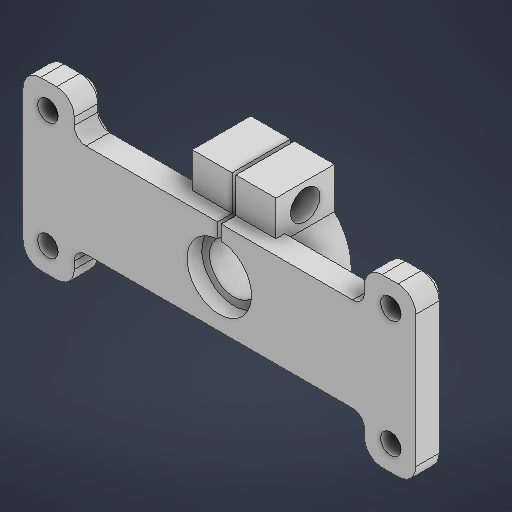
# Autodesk Inventor part: EndEffector_Holder_TEST
Saved by Autodesk Inventor 2025.2 (Build 292293000, 293)
## iProperties
Created: 2025-07-03
Part Number: EndEffector_Holder_TEST
Material: Generic
Document SubType Name: Modeling
Designer: Tiago
Density: 1 g/cm^3
Appearance: Default
Author: Tiago
Autodesk Inventor part; units mm, degrees
note: some values were not read from the file. Chosen so that the rebuilt part matches the saved one: sides of "Extrusion4".
ref_plane "YZ Plane" through (0, 0, 0) normal (1, 0, 0) x (0, 1, 0)
ref_plane "XZ Plane" through (0, 0, 0) normal (0, 1, 0) x (-1, 0, 0)
ref_plane "XY Plane" through (0, 0, 0) normal (0, 0, 1) x (1, 0, 0)
sketch "Sketch1" plane through (0, 0, 0) normal (0, 0, 1) x (1, 0, 0)
  line L0 (33.5, -11.25) -> (33.5, 11.25)
  line L1 (-33.5, 11.25) -> (-33.5, -11.25)
  circle A0 centre (-29.25, 10) radius 1.75
  circle A1 centre (29.25, 10) radius 1.75
  circle A2 centre (-29.25, -10) radius 1.75
  circle A3 centre (29.25, -10) radius 1.75
  circle A4 centre (0, 0) radius 5.5
  arc A5 (-30.5, 14.25) -> (-33.5, 11.25) centre (-30.5, 11.25) ccw
  arc A6 (-33.5, -11.25) -> (-30.5, -14.25) centre (-30.5, -11.25) ccw
  arc A7 (30.5, -14.25) -> (33.5, -11.25) centre (30.5, -11.25) ccw
  arc A8 (33.5, 11.25) -> (30.5, 14.25) centre (30.5, 11.25) ccw
  line L2 (-24.75, 10) -> (-24.75, 11.25)
  line L3 (24.75, 10) -> (24.75, 11.25)
  line L4 (30.5, 14.25) -> (27.75, 14.25)
  line L5 (-27.75, 14.25) -> (-30.5, 14.25)
  line L6 (-30.5, -14.25) -> (-27.75, -14.25)
  line L7 (27.75, -14.25) -> (30.5, -14.25)
  arc A9 (27.75, 14.25) -> (24.75, 11.25) centre (27.75, 11.25) ccw
  arc A10 (24.75, -11.25) -> (27.75, -14.25) centre (27.75, -11.25) ccw
  arc A11 (-27.75, -14.25) -> (-24.75, -11.25) centre (-27.75, -11.25) ccw
  arc A12 (-24.75, 11.25) -> (-27.75, 14.25) centre (-27.75, 11.25) ccw
  circle A13 centre (0, 0) radius 4.2
  line L8 (0, 0) -> (0, 1.4867) construction
  line L9 (-22.75, 8) -> (22.75, 8)
  line L10 (-22.75, -8) -> (22.75, -8)
  arc A14 (22.75, 8) -> (24.75, 10) centre (22.75, 10) ccw
  arc A15 (-24.75, 10) -> (-22.75, 8) centre (-22.75, 10) ccw
  line L11 (-24.75, -11.25) -> (-24.75, -10)
  line L12 (24.75, -11.25) -> (24.75, -10)
  arc A16 (24.75, -10) -> (22.75, -8) centre (22.75, -10) ccw
  arc A17 (-22.75, -8) -> (-24.75, -10) centre (-22.75, -10) ccw
  point P0 (-33.5, 0)
  point P1 (33.5, 0)
  point P2 (-24.75, -8)
  point P3 (24.75, -8)
  dimension "d0" = 58.5
  dimension "d1" = 3.5
  dimension "d2" = 3.5
  dimension "d3" = 20
  dimension "FF" = 3.5
  dimension "d5" = 3.5
  dimension "d7" = 67
  dimension "d8" = 29.25
  dimension "d9" = 10
  dimension "d10" = 11
  dimension "d11" = 3
  dimension "d12" = 4.5
  dimension "d13" = 4.5
  dimension "d14" = 3
  dimension "d15" = 33.5
  dimension "d16" = 28.5
  dimension "d17" = 8.4
  dimension "d27" = 2.5
  dimension "d28" = 8
  dimension "d29" = 2
  dimension "d30" = 2
  constraints: 28 tangent, 26 end point, 24 point on circle, 18 centre point, 9 perpendicular, 8 equal radius, 8 point on line, 5 horizontal alignment, 5 parallel, 2 coincident, 2 horizontal, 2 midpoint, 2 vertical, 2 vertical alignment
  measures "d0" distance of A1.centre A0.centre
  measures "d1" diameter of A1
  measures "d2" diameter of A0
  measures "d3" distance of A0.centre A2.centre
  measures "FF" diameter of A2
  measures "d5" diameter of A3
  measures "d7" distance between parallel lines of L0 L1
  measures "d8" horizontal distance of point (0, 0) A1.centre
  measures "d9" vertical distance of point (0, 0) A1.centre
  measures "d10" diameter of A4
  measures "d11" radius of A5
  measures "d12" distance from line of A2.centre L2
  measures "d13" distance from line of A1.centre L3
  measures "d14" radius of A9
  measures "d15" distance from line of point (0, 0) L0
  measures "d16" distance between parallel lines of L7 L4
  measures "d17" diameter of A13
  measures "d27" distance edge to line of A4 L10
  measures "d28" distance from line of L9 point (0, 0)
  measures "d29" radius of A14
  measures "d30" radius of A16
extrude "Extrusion1" add sketch "Sketch1" along normal blind 5 contours A7 L7 A10 L12 A16 L10 A17 L11 A11 L6 A6 L1 A5 L5 A12 L2 A15 L9 A14 L3 A9 L4 A8 L0
extrude "Extrusion2" add sketch "Sketch1" along normal blind 2.5 contours A4
sketch "Sketch2" plane through (0, 0, 0) normal (0, 0, -1) x (-1, 0, 0)
  circle A0 centre (0, 0) radius 4.2
  circle A1 centre (0, 0) radius 10
  line L0 (0, -10) -> (0, 14) construction
  line L1 (0, 14) -> (0, 9.5) construction
  line L2 (0, 9.5) -> (3.1225, 9.5) construction
  line L3 (3.1225, 7) -> (3.1225, 12)
  line L4 (3.1225, 12) -> (3.1225, 14)
  line L5 (3.1225, 14) -> (0, 14) construction
  line L6 (3.1225, 7) -> (7.1414, 7)
  line L7 (7.1414, 7) -> (7.1414, 10.0963)
  line L8 (7.1414, 10.0963) -> (3.1225, 10.0963)
  line L9 (3.1225, 9.5) -> (0.3225, 9.5) construction
  line L10 (0.3225, 9.5) -> (0.3225, 14)
  line L11 (0.3225, 14) -> (3.1225, 14)
  line L12 (3.1225, 14) -> (3.1225, 13)
  line L13 (3.1225, 7) -> (3.1225, 8)
  line L14 (3.1225, 8) -> (3.1225, 10.5)
  line L15 (-6.8775, 10.5) -> (13.1225, 10.5)
  line L16 (3.1225, 13) -> (0.3225, 13)
  line L17 (3.1225, 8) -> (0.3225, 8)
  line L18 (0.3225, 8) -> (0.3225, 9.5)
  line L19 (-3.1225, 8) -> (-0.3225, 8)
  line L20 (-3.1225, 8) -> (-3.1225, 10.5)
  line L21 (-3.1225, 7) -> (-3.1225, 12)
  line L22 (-3.1225, 7) -> (-7.1414, 7)
  line L23 (-7.1414, 7) -> (-7.1414, 10.0963)
  line L24 (-7.1414, 10.0963) -> (-3.1225, 10.0963)
  line L25 (-3.1225, 9.5) -> (-0.3225, 9.5) construction
  line L26 (-0.3225, 9.5) -> (-0.3225, 14)
  line L27 (-0.3225, 8) -> (-0.3225, 9.5)
  line L28 (-0.3225, 14) -> (-3.1225, 14)
  line L29 (-3.1225, 13) -> (-0.3225, 13)
  line L30 (-3.1225, 12) -> (-3.1225, 14)
  line L31 (-3.1225, 14) -> (-3.1225, 13)
  line L32 (3.1225, 7) -> (0.3225, 7)
  line L33 (0.3225, 7) -> (0.3225, 8)
  line L34 (-3.1225, 7) -> (-0.3225, 7)
  line L35 (-0.3225, 7) -> (-0.3225, 8)
  line L36 (-0.3225, 7) -> (-0.3225, 4.1876)
  line L37 (0.3225, 7) -> (0.3225, 4.1876)
  line L38 (7.1414, 7) -> (11.6713, 7)
  line L39 (-7.1414, 7) -> (-11.6713, 7)
  line L40 (-2.8125, 9.5963) -> (-3.1225, 5.975)
  line L41 (7.1414, 10.0963) -> (7.1414, 14)
  line L42 (3.1225, 14) -> (7.1414, 14)
  line L43 (-3.1225, 14) -> (-7.1414, 14)
  line L44 (-7.1414, 14) -> (-7.1414, 10.0963)
  line L45 (22.75, -8) -> (-22.75, -8) projected
  line L46 (-6, -8) -> (6, -8)
  point P0 (2.8125, 9.5963)
  point P1 (3.1225, 9.5055)
  point P2 (3.1225, 9.5)
  point P3 (0.3225, 9.9948)
  point P4 (-0.3225, 9.9948)
  dimension "d35" = 8.4
  dimension "d36" = 20
  dimension "d37" = 24
  dimension "d38" = 4.5
  dimension "d39" = 5
  dimension "d40" = 2.8
  dimension "d41" = 1
  dimension "d42" = 1
  dimension "d43" = 2.5
  dimension "d44" = 20
  constraints: 92 end point, 19 point on line, 15 symmetric about line, 11 perpendicular, 8 point on circle, 6 vertical, 4 midpoint, 3 coincident, 3 horizontal, 2 centre point, 1 collinear, 1 parallel
  measures "d35" diameter of A0
  measures "d36" diameter of A1
  measures "d37" distance of L0.start L0.end
  measures "d38" distance of L0.end L1.end
  measures "d39" distance of L6.start L3.end
  measures "d40" distance of L2.end L18.end
  measures "d41" distance of L42.start L12.end
  measures "d42" distance of L6.start L13.end
  measures "d43" distance of L13.end L14.end
  measures "d44" distance of L15.start L15.end
extrude "Extrusion3" add sketch "Sketch2" along normal blind 7.5 and the other way blind 2.5 contours A0 L37 L32 L6 A1 L45 L22 L34 L36 | L33 L17 L3 L32 | L34 L40 L19 L35 | L3 A1 L6 | L18 L10 A1 L3 L17 | L34 L21 L19 L40 | L19 L40 A1 L26 L27 | A1 L3 L8 L7 | L22 A1 L20 L21 | L19 L20 A1 L40 | A1 L10 L15 L3 | L8 L3 L15 L41 | L23 L24 L20 A1 | A1 L20 L15 L26 | L15 L3 L4 L42 L41 | L10 L16 L4 L3 L15 | L44 L43 L30 L21 L20 L24 | L15 L21 L30 L29 L26 | L10 L11 L4 L16 | L29 L30 L28 L26
extrude "Extrusion4" cut sketch "Sketch2" against normal through all both and the other way through all contours A0 L36 L35 L27 L26 A1 L10 L18 L33 L37
fillet "Fillet1" radius 5 2 edges at (-6, -8, -3.75) (6, -8, -3.75)
sketch "Sketch3" plane through (-7.1414, 7, 0) normal (-1, 0, 0) x (0, 0, 1)
  circle A0 centre (-2.5, 3.5) radius 2.5
  line L0 (2.5, 7) -> (-7.5, 7) projected
  line L1 (-7.5, 0) -> (-7.5, 7) projected
  point P0 (0, -7)
  dimension "d52" = 5
  dimension "d53" = 3.5
  dimension "d54" = 5
  constraints: 1 centre point
  measures "d52" diameter of A0
  measures "d53" distance from line of L0 A0.centre
  measures "d54" distance from line of L1 A0.centre
chamfer "Chamfer1" distance 1 angle 45 14 edges at (-14.9457, 8, 0) (-24.1642, 8.5858, 0) (-24.75, 10.625, 0) (-25.6287, 13.3713, 0) (-29.125, 14.25, 0) (-32.6213, 13.3713, 0) (-33.5, 0, 0) (-32.6213, -13.3713, 0) (-29.125, -14.25, 0) (-25.6287, -13.3713, 0) (-24.75, -10.625, 0) (-24.1642, -8.5858, 0) (-5, -8, 0) (-14.375, -8, 0)
chamfer "Chamfer2" distance 1 angle 45 14 edges at (14.375, -8, 0) (5, -8, 0) (24.1642, -8.5858, 0) (24.75, -10.625, 0) (25.6287, -13.3713, 0) (29.125, -14.25, 0) (32.6213, -13.3713, 0) (33.5, 0, 0) (32.6213, 13.3713, 0) (29.125, 14.25, 0) (25.6287, 13.3713, 0) (24.75, 10.625, 0) (24.1642, 8.5858, 0) (14.9457, 8, 0)
extrude "Extrusion5" cut sketch "Sketch3" against normal up to surface (14.2829 mm away)
chamfer "Chamfer3" distance 0.5 angle 45 1 edges at (0, -4.2, -7.5)
equation "\"d1\" = FF"
equation "\"d2\" = FF"
equation "\"d5\" = FF"
body "Solid1"
